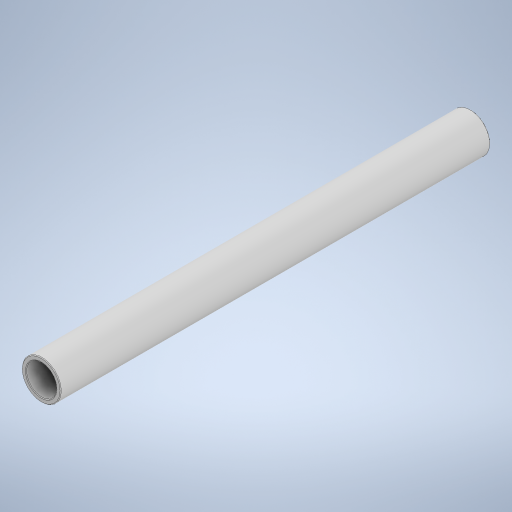
# Autodesk Inventor part: 筆桿
Saved by Autodesk Inventor 2024.2 (Build 282272000, 272)
## iProperties
Created: 2024-04-18
Part Number: 筆桿
Material: 一般
Document SubType Name: Modeling
Designer: User
Density: 1 g/cm^3
Appearance: 預設
Author: User
Autodesk Inventor part; units mm, degrees
ref_plane "YZ Plane" through (0, 0, 0) normal (1, 0, 0) x (0, 1, 0)
ref_plane "XZ Plane" through (0, 0, 0) normal (0, 1, 0) x (-1, 0, 0)
ref_plane "XY Plane" through (0, 0, 0) normal (0, 0, 1) x (1, 0, 0)
sketch "草圖1" plane through (0, 0, 0) normal (0, 1, 0) x (-1, 0, 0)
  line L0 (0, 0) -> (0, -99)
  line L1 (0, -99) -> (4.5, -99)
  line L2 (4.5, -99) -> (4.5, 0)
  line L3 (4.5, 0) -> (0, 0)
  line L4 (0, -99) -> (0, -81.5)
  line L5 (0, -81.5) -> (4.5, -81.5)
  dimension "d0" = 99
  dimension "d1" = 4.5
  dimension "d2" = 90
  dimension "d4" = 17.5
  constraints: 12 end point, 3 perpendicular, 2 point on line, 2 vertical
  measures "d0" distance of L0.start L0.end
  measures "d1" distance of L0.end L1.end
  measures "d2" angle of L1 L0
  measures "d4" distance of L0.end L4.end
revolve "迴轉3" add sketch "草圖1" angle 360 about axis through (-4.5, 0, -99) along (0, 0, 1) contours L3 L2 L5 L0
sketch "草圖3" plane through (-4.5, 0, -81.5) normal (0, 0, -1) x (-1, 0, 0)
  point P0 (-4.5, 0)
  point P1 (-0.0147, -0.0564)
hole "孔2" at (-4.4853, -0.0564, -81.5) direction (0, 0, 1) diameter 5 depth 66.5 tip angle 118
sketch "草圖4" plane through (-4.5, 0, 0) normal (0, 0, 1) x (1, 0, 0)
  point P0 (4.5, 0)
  point P1 (-0.0009, 0.0083)
hole "孔3" at (-4.5009, 0.0083, 0) direction (0, 0, -1) diameter 7 depth 15 tip angle 118
sketch "草圖5" plane through (-4.5, 0, -81.5) normal (0, 0, -1) x (-1, 0, 0)
  circle A0 centre (0, 0) radius 4.5
  point P0 (-4.5, 0)
  constraints: 1 centre point
extrude "擠出1" add sketch "草圖5" along normal blind 17.5
sketch "草圖6" plane through (-4.5, 0, -99) normal (0, 0, -1) x (-1, 0, 0)
  point P0 (-4.5, 0)
  point P1 (-0.0069, -0.0273)
hole "孔4" at (-4.4931, -0.0273, -99) direction (0, 0, 1) diameter 7 depth 17.5 tip angle 118
fillet "圓角1" radius 0.15 1 edges at (-9, 0, 0)
fillet "圓角2" radius 0.15 3 edges at (-4.5009, 3.5083, 0) (-4.4931, -3.5273, -99) (0, 0, -99)
